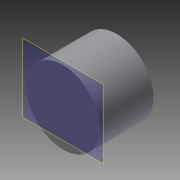
# Autodesk Inventor part: Part3
Saved by Autodesk Inventor 2014 SP1 (Build 180222100, 222)
## iProperties
Created: 2014-03-25
Part Number: Part3
Material: Generic
Document SubType Name: Modeling
Designer: tom
Density: 1 g/cm^3
Appearance: Default
Author: tom
Autodesk Inventor part; units mm, degrees
ref_plane "YZ Plane" through (0, 0, 0) normal (1, 0, 0) x (0, 1, 0)
ref_plane "XZ Plane" through (0, 0, 0) normal (0, 1, 0) x (-1, 0, 0)
ref_plane "XY Plane" through (0, 0, 0) normal (0, 0, 1) x (1, 0, 0)
ref_plane "Work Plane1" through (-21.7307, -25.2733, 26.6925) normal (0, 0, -1) x (-1, 0, 0)
sketch "Sketch1" plane through (-21.7307, -25.2733, 26.6925) normal (0, 0, -1) x (-1, 0, 0)
  circle A0 centre (7.5, 5.25) radius 1.5 projected
  line L0 (15, 0) -> (0, 0) projected
  line L1 (15, 0) -> (15, 5.25) projected
  arc A1 (15, 5.25) -> (0, 5.25) centre (7.5, 5.25) ccw projected
  line L2 (0, 0) -> (0, 5.25) projected
  circle A2 centre (7.5, 5.25) radius 7.5
  point P0 (-21.7307, 25.2733)
  constraints: 1 centre point, 1 coincident
extrude "Extrusion1" add sketch "Sketch1" along normal blind 11 contours A0 | A2 L0 | L0 A2 A1
body "Solid1"
